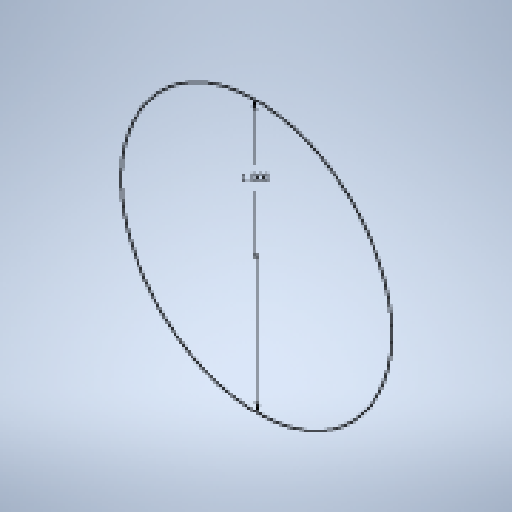
# Autodesk Inventor part: BasePlateMotorMount
Saved by Autodesk Inventor 2023 (Build 270158030, 158C)
## iProperties
Created: 2024-09-27
Part Number: BasePlateMotorMount
Material: Generic
Document SubType Name: Modeling
Designer: lvrectanus0
Density: 1 g/cm^3
Appearance: Default
Author: lvrectanus0
Autodesk Inventor part; units mm, degrees
(part 1 of 2)
ref_plane "YZ Plane" through (0, 0, 0) normal (1, 0, 0) x (0, 1, 0)
ref_plane "XZ Plane" through (0, 0, 0) normal (0, 1, 0) x (-1, 0, 0)
ref_plane "Work Plane1" through (-0.3933, 42.4252, 1.27) normal (0, 0, 1) x (1, 0, 0)
sketch "Sketch2" plane through (-0.3933, 42.4252, 1.27) normal (0, 0, 1) x (1, 0, 0)
  circle A0 centre (0.3933, -42.4252) radius 13.97 projected
  arc A1 (0.495, -45.4235) -> (0.2916, -45.4235) centre (0.3933, -42.4252) ccw projected
  line L0 (0.2916, -45.4235) -> (0.495, -45.4235) projected
  arc A2 (-5.2339, -23.0564) -> (-5.3005, -26.6101) centre (8.4164, -25.0898) ccw projected
  arc A3 (-5.3005, -26.6101) -> (-6.2823, -26.9988) centre (0.3933, -42.4252) ccw projected
  arc A4 (-6.2823, -26.9988) -> (-8.7636, -24.4539) centre (-17.3222, -35.2804) ccw projected
  arc A5 (-8.7636, -24.4539) -> (-9.8739, -25.0643) centre (0.3933, -42.4252) ccw projected
  arc A6 (-9.8739, -25.0643) -> (-9.0547, -28.5229) centre (3.8531, -23.6391) ccw projected
  arc A7 (-9.0547, -28.5229) -> (-9.909, -29.1436) centre (0.3933, -42.4252) ccw projected
  arc A8 (-9.909, -29.1436) -> (-12.9452, -27.2957) centre (-18.5425, -39.9105) ccw projected
  arc A9 (-12.9452, -27.2957) -> (-13.8688, -28.1631) centre (0.3933, -42.4252) ccw projected
  arc A10 (-13.8688, -28.1631) -> (-12.2152, -31.3093) centre (-0.9275, -23.3689) ccw projected
  arc A11 (-12.2152, -31.3093) -> (-12.8883, -32.1229) centre (0.3933, -42.4252) ccw projected
  arc A12 (-12.8883, -32.1229) -> (-16.2887, -31.0882) centre (-18.5729, -44.6986) ccw projected
  arc A13 (-16.2887, -31.0882) -> (-16.9676, -32.158) centre (0.3933, -42.4252) ccw projected
  arc A14 (-16.9676, -32.158) -> (-14.5835, -34.7941) centre (-5.6251, -24.296) ccw projected
  arc A15 (-14.5835, -34.7941) -> (-15.0331, -35.7496) centre (0.3933, -42.4252) ccw projected
  arc A16 (-15.0331, -35.7496) -> (-18.584, -35.593) centre (-17.4117, -49.3439) ccw projected
  arc A17 (-18.584, -35.593) -> (-18.9755, -36.798) centre (0.3933, -42.4252) ccw projected
  arc A18 (-18.9755, -36.798) -> (-16.0107, -38.7585) centre (-9.9445, -26.3623) ccw projected
  arc A19 (-16.0107, -38.7585) -> (-16.2086, -39.7957) centre (0.3933, -42.4252) ccw projected
  arc A20 (-16.2086, -39.7957) -> (-19.6869, -40.5271) centre (-15.1317, -53.5545) ccw projected
  arc A21 (-19.6869, -40.5271) -> (-19.7664, -41.7916) centre (0.3933, -42.4252) ccw projected
  arc A22 (-19.7664, -41.7916) -> (-16.4072, -42.9532) centre (-13.6144, -29.4379) ccw projected
  arc A23 (-16.4072, -42.9532) -> (-16.3409, -44.007) centre (0.3933, -42.4252) ccw projected
  arc A24 (-16.3409, -44.007) -> (-19.5281, -45.5804) centre (-11.8762, -57.0657) ccw projected
  arc A25 (-19.5281, -45.5804) -> (-19.2906, -46.8251) centre (0.3933, -42.4252) ccw projected
  arc A26 (-19.2906, -46.8251) -> (-15.7481, -47.1147) centre (-16.4042, -33.3295) ccw projected
  arc A27 (-15.7481, -47.1147) -> (-15.4218, -48.119) centre (0.3933, -42.4252) ccw projected
  arc A28 (-15.4218, -48.119) -> (-18.1175, -50.4355) centre (-7.8498, -59.6571) ccw projected
  arc A29 (-18.1175, -50.4355) -> (-17.578, -51.582) centre (0.3933, -42.4252) ccw projected
  arc A30 (-17.578, -51.582) -> (-14.0748, -50.9816) centre (-18.1385, -37.7926) ccw projected
  arc A31 (-14.0748, -50.9816) -> (-13.509, -51.8732) centre (0.3933, -42.4252) ccw projected
  arc A32 (-13.509, -51.8732) -> (-15.5439, -54.7873) centre (-3.3054, -61.1657) ccw projected
  arc A33 (-15.5439, -54.7873) -> (-14.7362, -55.7636) centre (0.3933, -42.4252) ccw projected
  arc A34 (-14.7362, -55.7636) -> (-11.4923, -54.3108) centre (-18.7083, -42.5468) ccw projected
  arc A35 (-11.4923, -54.3108) -> (-10.7226, -55.0337) centre (0.3933, -42.4252) ccw projected
  arc A36 (-10.7226, -55.0337) -> (-11.9689, -58.3624) centre (1.4713, -61.4968) ccw projected
  arc A37 (-11.9689, -58.3624) -> (-10.9438, -59.1071) centre (0.3933, -42.4252) ccw projected
  arc A38 (-10.9438, -59.1071) -> (-8.1631, -56.8933) centre (-18.078, -47.2933) ccw projected
  arc A39 (-8.1631, -56.8933) -> (-7.2378, -57.402) centre (0.3933, -42.4252) ccw projected
  arc A40 (-7.2378, -57.402) -> (-7.6171, -60.936) centre (6.1804, -60.6295) ccw projected
  arc A41 (-7.6171, -60.936) -> (-6.439, -61.4025) centre (0.3933, -42.4252) ccw projected
  arc A42 (-6.439, -61.4025) -> (-4.2962, -58.5666) centre (-16.287, -51.734) ccw projected
  arc A43 (-4.2962, -58.5666) -> (-3.2734, -58.8292) centre (0.3933, -42.4252) ccw projected
  arc A44 (-3.2734, -58.8292) -> (-2.7619, -62.3466) centre (10.5258, -58.6184) ccw projected
  arc A45 (-2.7619, -62.3466) -> (-1.5049, -62.5054) centre (0.3933, -42.4252) ccw projected
  arc A46 (-1.5049, -62.5054) -> (-0.1347, -59.2257) centre (-13.448, -55.5898) ccw projected
  arc A47 (-0.1347, -59.2257) -> (0.9213, -59.2257) centre (0.3933, -42.4252) ccw projected
  arc A48 (0.9213, -59.2257) -> (2.2914, -62.5054) centre (14.2345, -55.5898) ccw projected
  arc A49 (2.2914, -62.5054) -> (3.5485, -62.3466) centre (0.3933, -42.4252) ccw projected
  arc A50 (3.5485, -62.3466) -> (4.06, -58.8292) centre (-9.7392, -58.6184) ccw projected
  arc A51 (4.06, -58.8292) -> (5.0828, -58.5666) centre (0.3933, -42.4252) ccw projected
  arc A52 (5.0828, -58.5666) -> (7.2255, -61.4025) centre (17.0736, -51.734) ccw projected
  arc A53 (7.2255, -61.4025) -> (8.4036, -60.936) centre (0.3933, -42.4252) ccw projected
  arc A54 (8.4036, -60.936) -> (8.0243, -57.402) centre (-5.3938, -60.6295) ccw projected
  arc A55 (8.0243, -57.402) -> (8.9497, -56.8933) centre (0.3933, -42.4252) ccw projected
  arc A56 (8.9497, -56.8933) -> (11.7303, -59.1071) centre (18.8646, -47.2933) ccw projected
  arc A57 (11.7303, -59.1071) -> (12.7554, -58.3624) centre (0.3933, -42.4252) ccw projected
  arc A58 (12.7554, -58.3624) -> (11.5092, -55.0337) centre (-0.6848, -61.4968) ccw projected
  arc A59 (11.5092, -55.0337) -> (12.2789, -54.3108) centre (0.3933, -42.4252) ccw projected
  arc A60 (12.2789, -54.3108) -> (15.5228, -55.7636) centre (19.4949, -42.5468) ccw projected
  arc A61 (15.5228, -55.7636) -> (16.3305, -54.7873) centre (0.3933, -42.4252) ccw projected
  arc A62 (16.3305, -54.7873) -> (14.2955, -51.8732) centre (4.092, -61.1657) ccw projected
  arc A63 (14.2955, -51.8732) -> (14.8613, -50.9816) centre (0.3933, -42.4252) ccw projected
  arc A64 (14.8613, -50.9816) -> (18.3646, -51.582) centre (18.925, -37.7926) ccw projected
  arc A65 (18.3646, -51.582) -> (18.9041, -50.4355) centre (0.3933, -42.4252) ccw projected
  arc A66 (18.9041, -50.4355) -> (16.2084, -48.119) centre (8.6364, -59.6571) ccw projected
  arc A67 (16.2084, -48.119) -> (16.5347, -47.1147) centre (0.3933, -42.4252) ccw projected
  arc A68 (16.5347, -47.1147) -> (20.0772, -46.8251) centre (17.1907, -33.3295) ccw projected
  arc A69 (20.0772, -46.8251) -> (20.3146, -45.5804) centre (0.3933, -42.4252) ccw projected
  arc A70 (20.3146, -45.5804) -> (17.1275, -44.007) centre (12.6628, -57.0657) ccw projected
  arc A71 (17.1275, -44.007) -> (17.1938, -42.9532) centre (0.3933, -42.4252) ccw projected
  arc A72 (17.1938, -42.9532) -> (20.553, -41.7916) centre (14.401, -29.4379) ccw projected
  arc A73 (20.553, -41.7916) -> (20.4735, -40.5271) centre (0.3933, -42.4252) ccw projected
  arc A74 (20.4735, -40.5271) -> (16.9952, -39.7957) centre (15.9183, -53.5545) ccw projected
  arc A75 (16.9952, -39.7957) -> (16.7973, -38.7585) centre (0.3933, -42.4252) ccw projected
  arc A76 (16.7973, -38.7585) -> (19.7621, -36.798) centre (10.7311, -26.3623) ccw projected
  arc A77 (19.7621, -36.798) -> (19.3706, -35.593) centre (0.3933, -42.4252) ccw projected
  arc A78 (19.3706, -35.593) -> (15.8197, -35.7496) centre (18.1983, -49.3439) ccw projected
  arc A79 (15.8197, -35.7496) -> (15.3701, -34.7941) centre (0.3933, -42.4252) ccw projected
  arc A80 (15.3701, -34.7941) -> (17.7542, -32.158) centre (6.4116, -24.296) ccw projected
  arc A81 (17.7542, -32.158) -> (17.0752, -31.0882) centre (0.3933, -42.4252) ccw projected
  arc A82 (17.0752, -31.0882) -> (13.6749, -32.1229) centre (19.3595, -44.6986) ccw projected
  arc A83 (13.6749, -32.1229) -> (13.0018, -31.3093) centre (0.3933, -42.4252) ccw projected
  arc A84 (13.0018, -31.3093) -> (14.6554, -28.1631) centre (1.714, -23.3689) ccw projected
  arc A85 (14.6554, -28.1631) -> (13.7317, -27.2957) centre (0.3933, -42.4252) ccw projected
  arc A86 (13.7317, -27.2957) -> (10.6955, -29.1436) centre (19.329, -39.9105) ccw projected
  arc A87 (10.6955, -29.1436) -> (9.8412, -28.5229) centre (0.3933, -42.4252) ccw projected
  arc A88 (9.8412, -28.5229) -> (10.6605, -25.0643) centre (-3.0666, -23.6391) ccw projected
  arc A89 (10.6605, -25.0643) -> (9.5501, -24.4539) centre (0.3933, -42.4252) ccw projected
  arc A90 (9.5501, -24.4539) -> (7.0689, -26.9988) centre (18.1088, -35.2804) ccw projected
  arc A91 (7.0689, -26.9988) -> (6.0871, -26.6101) centre (0.3933, -42.4252) ccw projected
  arc A92 (6.0871, -26.6101) -> (6.0204, -23.0564) centre (-7.6298, -25.0898) ccw projected
  arc A93 (6.0204, -23.0564) -> (4.7932, -22.7413) centre (0.3933, -42.4252) ccw projected
  arc A94 (4.7932, -22.7413) -> (3.0228, -25.8233) centre (15.7754, -31.0992) ccw projected
  arc A95 (3.0228, -25.8233) -> (1.9751, -25.691) centre (0.3933, -42.4252) ccw projected
  arc A96 (1.9751, -25.691) -> (1.0268, -22.2655) centre (-11.6889, -27.6297) ccw projected
  arc A97 (1.0268, -22.2655) -> (-0.2403, -22.2655) centre (0.3933, -42.4252) ccw projected
  arc A98 (-0.2403, -22.2655) -> (-1.1886, -25.691) centre (12.4754, -27.6297) ccw projected
  arc A99 (-1.1886, -25.691) -> (-2.2362, -25.8233) centre (0.3933, -42.4252) ccw projected
  arc A100 (-2.2362, -25.8233) -> (-4.0066, -22.7413) centre (-14.9888, -31.0992) ccw projected
  arc A101 (-4.0066, -22.7413) -> (-5.2339, -23.0564) centre (0.3933, -42.4252) ccw projected
  arc A102 (3.4869, -25.0828) -> (4.2324, -21.6038) centre (-12.0318, -19.9381) ccw projected
  arc A103 (4.2324, -21.6038) -> (5.318, -21.4226) centre (0.3933, 4.7462) ccw projected
  arc A104 (5.318, -21.4226) -> (7.1528, -24.4711) centre (20.1601, -14.5662) ccw projected
  arc A105 (7.1528, -24.4711) -> (8.3544, -24.1668) centre (0.3933, 4.7462) ccw projected
  arc A106 (8.3544, -24.1668) -> (8.5171, -20.6125) centre (-7.7994, -21.6465) ccw projected
  arc A107 (8.5171, -20.6125) -> (9.5581, -20.2551) centre (0.3933, 4.7462) ccw projected
  arc A108 (9.5581, -20.2551) -> (11.8696, -22.9601) centre (23.0692, -11.0493) ccw projected
  arc A109 (11.8696, -22.9601) -> (13.0048, -22.4621) centre (0.3933, 4.7462) ccw projected
  arc A110 (13.0048, -22.4621) -> (12.5802, -18.9295) centre (-3.3436, -22.6351) ccw projected
  arc A111 (12.5802, -18.9295) -> (13.5482, -18.4057) centre (0.3933, 4.7462) ccw projected
  arc A112 (13.5482, -18.4057) -> (16.2734, -20.6932) centre (25.3598, -7.1016) ccw projected
  arc A113 (16.2734, -20.6932) -> (17.3111, -20.0153) centre (0.3933, 4.7462) ccw projected
  arc A114 (17.3111, -20.0153) -> (16.3109, -16.6007) centre (1.2142, -22.8767) ccw projected
  arc A115 (16.3109, -16.6007) -> (17.1795, -15.9247) centre (0.3933, 4.7462) ccw projected
  arc A116 (17.1795, -15.9247) -> (20.244, -17.7325) centre (26.9694, -2.8306) ccw projected
  arc A117 (20.244, -17.7325) -> (21.156, -16.893) centre (0.3933, 4.7462) ccw projected
  arc A118 (21.156, -16.893) -> (19.6074, -13.6896) centre (5.7496, -22.3648) ccw projected
  arc A119 (19.6074, -13.6896) -> (20.3528, -12.8798) centre (0.3933, 4.7462) ccw projected
  arc A120 (20.3528, -12.8798) -> (23.6731, -14.1586) centre (27.854, 1.647) ccw projected
  arc A121 (23.6731, -14.1586) -> (24.4345, -13.1804) centre (0.3933, 4.7462) ccw projected
  arc A122 (24.4345, -13.1804) -> (22.3798, -10.2756) centre (10.1389, -21.1134) ccw projected
  arc A123 (22.3798, -10.2756) -> (22.9818, -9.3542) centre (0.3933, 4.7462) ccw projected
  arc A124 (22.9818, -9.3542) -> (26.4673, -10.069) centre (27.9896, 6.2092) ccw projected
  arc A125 (26.4673, -10.069) -> (27.0572, -8.9789) centre (0.3933, 4.7462) ccw projected
  arc A126 (27.0572, -8.9789) -> (24.5524, -6.4519) centre (14.2623, -19.1567) ccw projected
  arc A127 (24.5524, -6.4519) -> (24.9945, -5.4439) centre (0.3933, 4.7462) ccw projected
  arc A128 (24.9945, -5.4439) -> (28.5502, -5.5753) centre (27.3725, 10.7314) ccw projected
  arc A129 (28.5502, -5.5753) -> (28.9527, -4.4029) centre (0.3933, 4.7462) ccw projected
  arc A130 (28.9527, -4.4029) -> (26.0661, -2.3227) centre (18.0075, -16.5479) ccw projected
  arc A131 (26.0661, -2.3227) -> (26.3363, -1.2557) centre (0.3933, 4.7462) ccw projected
  arc A132 (26.3363, -1.2557) -> (29.865, -0.8001) centre (26.0194, 15.0904) ccw projected
  arc A133 (29.865, -0.8001) -> (30.069, 0.4226) centre (0.3933, 4.7462) ccw projected
  arc A134 (30.069, 0.4226) -> (26.8794, 1.9993) centre (21.2721, -13.3583) ccw projected
  arc A135 (26.8794, 1.9993) -> (26.9703, 3.0962) centre (0.3933, 4.7462) ccw projected
  arc A136 (26.9703, 3.0962) -> (30.376, 4.1265) centre (23.9673, 19.1673) ccw projected
  arc A137 (30.376, 4.1265) -> (30.376, 5.366) centre (0.3933, 4.7462) ccw projected
  arc A138 (30.376, 5.366) -> (26.9703, 6.3963) centre (23.9673, -9.6748) ccw projected
  arc A139 (26.9703, 6.3963) -> (26.8794, 7.4931) centre (0.3933, 4.7462) ccw projected
  arc A140 (26.8794, 7.4931) -> (30.069, 9.0699) centre (21.2721, 22.8507) ccw projected
  arc A141 (30.069, 9.0699) -> (29.865, 10.2925) centre (0.3933, 4.7462) ccw projected
  arc A142 (29.865, 10.2925) -> (26.3363, 10.7482) centre (26.0194, -5.598) ccw projected
  arc A143 (26.3363, 10.7482) -> (26.0661, 11.8152) centre (0.3933, 4.7462) ccw projected
  arc A144 (26.0661, 11.8152) -> (28.9527, 13.8954) centre (18.0075, 26.0404) ccw projected
  arc A145 (28.9527, 13.8954) -> (28.5502, 15.0678) centre (0.3933, 4.7462) ccw projected
  arc A146 (28.5502, 15.0678) -> (24.9945, 14.9364) centre (27.3725, -1.239) ccw projected
  arc A147 (24.9945, 14.9364) -> (24.5524, 15.9444) centre (0.3933, 4.7462) ccw projected
  arc A148 (24.5524, 15.9444) -> (27.0572, 18.4713) centre (14.2623, 28.6491) ccw projected
  arc A149 (27.0572, 18.4713) -> (26.4673, 19.5615) centre (0.3933, 4.7462) ccw projected
  arc A150 (26.4673, 19.5615) -> (22.9818, 18.8467) centre (27.9896, 3.2833) ccw projected
  arc A151 (22.9818, 18.8467) -> (22.3798, 19.7681) centre (0.3933, 4.7462) ccw projected
  arc A152 (22.3798, 19.7681) -> (24.4345, 22.6729) centre (10.1389, 30.6059) ccw projected
  arc A153 (24.4345, 22.6729) -> (23.6731, 23.6511) centre (0.3933, 4.7462) ccw projected
  arc A154 (23.6731, 23.6511) -> (20.3528, 22.3723) centre (27.854, 7.8455) ccw projected
  arc A155 (20.3528, 22.3723) -> (19.6074, 23.1821) centre (0.3933, 4.7462) ccw projected
  arc A156 (19.6074, 23.1821) -> (21.156, 26.3854) centre (5.7496, 31.8573) ccw projected
  arc A157 (21.156, 26.3854) -> (20.244, 27.225) centre (0.3933, 4.7462) ccw projected
  arc A158 (20.244, 27.225) -> (17.1795, 25.4171) centre (26.9694, 12.3231) ccw projected
  arc A159 (17.1795, 25.4171) -> (16.3109, 26.0932) centre (0.3933, 4.7462) ccw projected
  arc A160 (16.3109, 26.0932) -> (17.3111, 29.5077) centre (1.2142, 32.3691) ccw projected
  arc A161 (17.3111, 29.5077) -> (16.2734, 30.1857) centre (0.3933, 4.7462) ccw projected
  arc A162 (16.2734, 30.1857) -> (13.5482, 27.8981) centre (25.3598, 16.594) ccw projected
  arc A163 (13.5482, 27.8981) -> (12.5802, 28.422) centre (0.3933, 4.7462) ccw projected
  arc A164 (12.5802, 28.422) -> (13.0048, 31.9546) centre (-3.3436, 32.1275) ccw projected
  arc A165 (13.0048, 31.9546) -> (11.8696, 32.4525) centre (0.3933, 4.7462) ccw projected
  arc A166 (11.8696, 32.4525) -> (9.5581, 29.7476) centre (23.0692, 20.5418) ccw projected
  arc A167 (9.5581, 29.7476) -> (8.5171, 30.105) centre (0.3933, 4.7462) ccw projected
  arc A168 (8.5171, 30.105) -> (8.3544, 33.6593) centre (-7.7994, 31.139) ccw projected
  arc A169 (8.3544, 33.6593) -> (7.1528, 33.9636) centre (0.3933, 4.7462) ccw projected
  arc A170 (7.1528, 33.9636) -> (5.318, 30.9151) centre (20.1601, 24.0587) ccw projected
  arc A171 (5.318, 30.9151) -> (4.2324, 31.0962) centre (0.3933, 4.7462) ccw projected
  arc A172 (4.2324, 31.0962) -> (3.4869, 34.5753) centre (-12.0318, 29.4306) ccw projected
  arc A173 (3.4869, 34.5753) -> (2.2516, 34.6777) centre (0.3933, 4.7462) ccw projected
  arc A174 (2.2516, 34.6777) -> (0.9436, 31.3688) centre (16.7118, 27.0488) ccw projected
  arc A175 (0.9436, 31.3688) -> (-0.157, 31.3688) centre (0.3933, 4.7462) ccw projected
  arc A176 (-0.157, 31.3688) -> (-1.465, 34.6777) centre (-15.9252, 27.0488) ccw projected
  arc A177 (-1.465, 34.6777) -> (-2.7003, 34.5753) centre (0.3933, 4.7462) ccw projected
  arc A178 (-2.7003, 34.5753) -> (-3.4458, 31.0962) centre (12.8183, 29.4306) ccw projected
  arc A179 (-3.4458, 31.0962) -> (-4.5315, 30.9151) centre (0.3933, 4.7462) ccw projected
  arc A180 (-4.5315, 30.9151) -> (-6.3662, 33.9636) centre (-19.3735, 24.0587) ccw projected
  arc A181 (-6.3662, 33.9636) -> (-7.5678, 33.6593) centre (0.3933, 4.7462) ccw projected
  arc A182 (-7.5678, 33.6593) -> (-7.7305, 30.105) centre (8.586, 31.139) ccw projected
  arc A183 (-7.7305, 30.105) -> (-8.7715, 29.7476) centre (0.3933, 4.7462) ccw projected
  arc A184 (-8.7715, 29.7476) -> (-11.083, 32.4525) centre (-22.2827, 20.5418) ccw projected
  arc A185 (-11.083, 32.4525) -> (-12.2182, 31.9546) centre (0.3933, 4.7462) ccw projected
  arc A186 (-12.2182, 31.9546) -> (-11.7936, 28.422) centre (4.1301, 32.1275) ccw projected
  arc A187 (-11.7936, 28.422) -> (-12.7616, 27.8981) centre (0.3933, 4.7462) ccw projected
  arc A188 (-12.7616, 27.8981) -> (-15.4868, 30.1857) centre (-24.5733, 16.594) ccw projected
  arc A189 (-15.4868, 30.1857) -> (-16.5245, 29.5077) centre (0.3933, 4.7462) ccw projected
  arc A190 (-16.5245, 29.5077) -> (-15.5243, 26.0932) centre (-0.4277, 32.3691) ccw projected
  arc A191 (-15.5243, 26.0932) -> (-16.3929, 25.4171) centre (0.3933, 4.7462) ccw projected
  arc A192 (-16.3929, 25.4171) -> (-19.4574, 27.225) centre (-26.1828, 12.3231) ccw projected
  arc A193 (-19.4574, 27.225) -> (-20.3694, 26.3854) centre (0.3933, 4.7462) ccw projected
  arc A194 (-20.3694, 26.3854) -> (-18.8208, 23.1821) centre (-4.963, 31.8573) ccw projected
  arc A195 (-18.8208, 23.1821) -> (-19.5663, 22.3723) centre (0.3933, 4.7462) ccw projected
  arc A196 (-19.5663, 22.3723) -> (-22.8866, 23.6511) centre (-27.0675, 7.8455) ccw projected
  arc A197 (-22.8866, 23.6511) -> (-23.6479, 22.6729) centre (0.3933, 4.7462) ccw projected
  arc A198 (-23.6479, 22.6729) -> (-21.5932, 19.7681) centre (-9.3523, 30.6059) ccw projected
  arc A199 (-21.5932, 19.7681) -> (-22.1952, 18.8467) centre (0.3933, 4.7462) ccw projected
  arc A200 (-22.1952, 18.8467) -> (-25.6807, 19.5615) centre (-27.2031, 3.2833) ccw projected
  arc A201 (-25.6807, 19.5615) -> (-26.2707, 18.4713) centre (0.3933, 4.7462) ccw projected
  arc A202 (-26.2707, 18.4713) -> (-23.7659, 15.9444) centre (-13.4758, 28.6491) ccw projected
  arc A203 (-23.7659, 15.9444) -> (-24.208, 14.9364) centre (0.3933, 4.7462) ccw projected
  arc A204 (-24.208, 14.9364) -> (-27.7636, 15.0678) centre (-26.5859, -1.239) ccw projected
  arc A205 (-27.7636, 15.0678) -> (-28.1661, 13.8954) centre (0.3933, 4.7462) ccw projected
  arc A206 (-28.1661, 13.8954) -> (-25.2795, 11.8152) centre (-17.2209, 26.0404) ccw projected
  arc A207 (-25.2795, 11.8152) -> (-25.5497, 10.7482) centre (0.3933, 4.7462) ccw projected
  arc A208 (-25.5497, 10.7482) -> (-29.0784, 10.2925) centre (-25.2328, -5.598) ccw projected
  arc A209 (-29.0784, 10.2925) -> (-29.2825, 9.0699) centre (0.3933, 4.7462) ccw projected
  arc A210 (-29.2825, 9.0699) -> (-26.0929, 7.4931) centre (-20.4856, 22.8507) ccw projected
  arc A211 (-26.0929, 7.4931) -> (-26.1838, 6.3963) centre (0.3933, 4.7462) ccw projected
  arc A212 (-26.1838, 6.3963) -> (-29.5894, 5.366) centre (-23.1807, -9.6748) ccw projected
  arc A213 (-29.5894, 5.366) -> (-29.5894, 4.1265) centre (0.3933, 4.7462) ccw projected
  arc A214 (-29.5894, 4.1265) -> (-26.1838, 3.0962) centre (-23.1807, 19.1673) ccw projected
  arc A215 (-26.1838, 3.0962) -> (-26.0929, 1.9993) centre (0.3933, 4.7462) ccw projected
  arc A216 (-26.0929, 1.9993) -> (-29.2825, 0.4226) centre (-20.4856, -13.3583) ccw projected
  arc A217 (-29.2825, 0.4226) -> (-29.0784, -0.8001) centre (0.3933, 4.7462) ccw projected
  arc A218 (-29.0784, -0.8001) -> (-25.5497, -1.2557) centre (-25.2328, 15.0904) ccw projected
  arc A219 (-25.5497, -1.2557) -> (-25.2795, -2.3227) centre (0.3933, 4.7462) ccw projected
  arc A220 (-25.2795, -2.3227) -> (-28.1661, -4.4029) centre (-17.2209, -16.5479) ccw projected
  arc A221 (-28.1661, -4.4029) -> (-27.7636, -5.5753) centre (0.3933, 4.7462) ccw projected
  arc A222 (-27.7636, -5.5753) -> (-24.208, -5.4439) centre (-26.5859, 10.7314) ccw projected
  arc A223 (-24.208, -5.4439) -> (-23.7659, -6.4519) centre (0.3933, 4.7462) ccw projected
  arc A224 (-23.7659, -6.4519) -> (-26.2707, -8.9789) centre (-13.4758, -19.1567) ccw projected
  arc A225 (-26.2707, -8.9789) -> (-25.6807, -10.069) centre (0.3933, 4.7462) ccw projected
  arc A226 (-25.6807, -10.069) -> (-22.1952, -9.3542) centre (-27.2031, 6.2092) ccw projected
  arc A227 (-22.1952, -9.3542) -> (-21.5932, -10.2756) centre (0.3933, 4.7462) ccw projected
  arc A228 (-21.5932, -10.2756) -> (-23.6479, -13.1804) centre (-9.3523, -21.1134) ccw projected
  arc A229 (-23.6479, -13.1804) -> (-22.8866, -14.1586) centre (0.3933, 4.7462) ccw projected
  arc A230 (-22.8866, -14.1586) -> (-19.5663, -12.8798) centre (-27.0675, 1.647) ccw projected
  arc A231 (-19.5663, -12.8798) -> (-18.8208, -13.6896) centre (0.3933, 4.7462) ccw projected
  arc A232 (-18.8208, -13.6896) -> (-20.3694, -16.893) centre (-4.963, -22.3648) ccw projected
  arc A233 (-20.3694, -16.893) -> (-19.4574, -17.7325) centre (0.3933, 4.7462) ccw projected
  arc A234 (-19.4574, -17.7325) -> (-16.3929, -15.9247) centre (-26.1828, -2.8306) ccw projected
  arc A235 (-16.3929, -15.9247) -> (-15.5243, -16.6007) centre (0.3933, 4.7462) ccw projected
  arc A236 (-15.5243, -16.6007) -> (-16.5245, -20.0153) centre (-0.4277, -22.8767) ccw projected
  arc A237 (-16.5245, -20.0153) -> (-15.4868, -20.6932) centre (0.3933, 4.7462) ccw projected
  arc A238 (-15.4868, -20.6932) -> (-12.7616, -18.4057) centre (-24.5733, -7.1016) ccw projected
  arc A239 (-12.7616, -18.4057) -> (-11.7936, -18.9295) centre (0.3933, 4.7462) ccw projected
  arc A240 (-11.7936, -18.9295) -> (-12.2182, -22.4621) centre (4.1301, -22.6351) ccw projected
  arc A241 (-12.2182, -22.4621) -> (-11.083, -22.9601) centre (0.3933, 4.7462) ccw projected
  arc A242 (-11.083, -22.9601) -> (-8.7715, -20.2551) centre (-22.2827, -11.0493) ccw projected
  arc A243 (-8.7715, -20.2551) -> (-7.7305, -20.6125) centre (0.3933, 4.7462) ccw projected
  arc A244 (-7.7305, -20.6125) -> (-7.5678, -24.1668) centre (8.586, -21.6465) ccw projected
  arc A245 (-7.5678, -24.1668) -> (-6.3662, -24.4711) centre (0.3933, 4.7462) ccw projected
  arc A246 (-6.3662, -24.4711) -> (-4.5315, -21.4226) centre (-19.3735, -14.5662) ccw projected
  arc A247 (-4.5315, -21.4226) -> (-3.4458, -21.6038) centre (0.3933, 4.7462) ccw projected
  arc A248 (-3.4458, -21.6038) -> (-2.7003, -25.0828) centre (12.8183, -19.9381) ccw projected
  arc A249 (-2.7003, -25.0828) -> (-1.465, -25.1852) centre (0.3933, 4.7462) ccw projected
  arc A250 (-1.465, -25.1852) -> (-0.157, -21.8763) centre (-15.9252, -17.5564) ccw projected
  arc A251 (-0.157, -21.8763) -> (0.9436, -21.8763) centre (0.3933, 4.7462) ccw projected
  arc A252 (0.9436, -21.8763) -> (2.2516, -25.1852) centre (16.7118, -17.5564) ccw projected
  arc A253 (2.2516, -25.1852) -> (3.4869, -25.0828) centre (0.3933, 4.7462) ccw projected
  line L1 (3.3661, -1.5533) -> (7.3352, 4.171) projected
  line L2 (-3.5758, -0.978) -> (3.3661, -1.5533) projected
  line L3 (-6.5487, 5.3215) -> (-3.5758, -0.978) projected
  line L4 (-2.5795, 11.0457) -> (-6.5487, 5.3215) projected
  line L5 (4.3624, 10.4705) -> (-2.5795, 11.0457) projected
  line L6 (7.3352, 4.171) -> (4.3624, 10.4705) projected
  arc A254 (5.8315, -120.0023) -> (6.7501, -116.5589) centre (-13.9026, -112.8937) ccw projected
  arc A255 (4.6244, -120.0775) -> (5.8315, -120.0023) centre (0.3933, -42.4252) ccw projected
  arc A256 (3.2855, -116.7747) -> (4.6244, -120.0775) centre (23.3237, -110.5748) ccw projected
  arc A257 (2.1289, -116.8107) -> (3.2855, -116.7747) centre (0.3933, -42.4252) ccw projected
  arc A258 (0.998, -120.1904) -> (2.1289, -116.8107) centre (-18.256, -111.8686) ccw projected
  arc A259 (-0.2114, -120.1904) -> (0.998, -120.1904) centre (0.3933, -42.4252) ccw projected
  arc A260 (-1.3423, -116.8107) -> (-0.2114, -120.1904) centre (19.0425, -111.8686) ccw projected
  arc A261 (-2.499, -116.7747) -> (-1.3423, -116.8107) centre (0.3933, -42.4252) ccw projected
  arc A262 (-3.8378, -120.0775) -> (-2.499, -116.7747) centre (-22.5371, -110.5748) ccw projected
  arc A263 (-5.0449, -120.0023) -> (-3.8378, -120.0775) centre (0.3933, -42.4252) ccw projected
  arc A264 (-5.9635, -116.5589) -> (-5.0449, -120.0023) centre (14.6892, -112.8937) ccw projected
  arc A265 (-7.1157, -116.4511) -> (-5.9635, -116.5589) centre (0.3933, -42.4252) ccw projected
  arc A266 (-8.6572, -119.6643) -> (-7.1157, -116.4511) centre (-26.7296, -109.0174) ccw projected
  arc A267 (-9.8573, -119.5142) -> (-8.6572, -119.6643) centre (0.3933, -42.4252) ccw projected
  arc A268 (-10.5601, -116.0203) -> (-9.8573, -119.5142) centre (10.2805, -113.6461) ccw projected
  arc A269 (-11.7033, -115.8411) -> (-10.5601, -116.0203) centre (0.3933, -42.4252) ccw projected
  arc A270 (-13.4416, -118.9522) -> (-11.7033, -115.8411) centre (-30.8172, -107.2024) ccw projected
  arc A271 (-14.6301, -118.7278) -> (-13.4416, -118.9522) centre (0.3933, -42.4252) ccw projected
  arc A272 (-15.1143, -115.197) -> (-14.6301, -118.7278) centre (5.8336, -114.123) ccw projected
  arc A273 (-16.2441, -114.947) -> (-15.1143, -115.197) centre (0.3933, -42.4252) ccw projected
  arc A274 (-18.1725, -117.944) -> (-16.2441, -114.947) centre (-34.784, -105.1367) ccw projected
  arc A275 (-19.3447, -117.6462) -> (-18.1725, -117.944) centre (0.3933, -42.4252) ccw projected
  arc A276 (-19.6085, -114.0921) -> (-19.3447, -117.6462) centre (1.3657, -114.3226) ccw projected
  arc A277 (-20.7206, -113.7724) -> (-19.6085, -114.0921) centre (0.3933, -42.4252) ccw projected
  arc A278 (-22.8316, -116.6437) -> (-20.7206, -113.7724) centre (-38.6147, -102.8285) ccw projected
  arc A279 (-23.983, -116.2736) -> (-22.8316, -116.6437) centre (0.3933, -42.4252) ccw projected
  arc A280 (-24.0253, -112.71) -> (-23.983, -116.2736) centre (-3.106, -114.2439) ccw projected
  arc A281 (-25.1154, -112.3217) -> (-24.0253, -112.71) centre (0.3933, -42.4252) ccw projected
  arc A282 (-27.4008, -115.0563) -> (-25.1154, -112.3217) centre (-42.2945, -100.2865) ccw projected
  arc A283 (-28.527, -114.6152) -> (-27.4008, -115.0563) centre (0.3933, -42.4252) ccw projected
  arc A284 (-28.3476, -111.0559) -> (-28.527, -114.6152) centre (-7.5642, -113.8875) ccw projected
  arc A285 (-29.4115, -110.6006) -> (-28.3476, -111.0559) centre (0.3933, -42.4252) ccw projected
  arc A286 (-31.8625, -113.1878) -> (-29.4115, -110.6006) centre (-45.8091, -97.5207) ccw projected
  arc A287 (-32.9591, -112.6776) -> (-31.8625, -113.1878) centre (0.3933, -42.4252) ccw projected
  arc A288 (-32.5588, -109.1363) -> (-32.9591, -112.6776) centre (-11.9916, -113.2545) ccw projected
  arc A289 (-33.5923, -108.6158) -> (-32.5588, -109.1363) centre (0.3933, -42.4252) ccw projected
  arc A290 (-36.1994, -111.0456) -> (-33.5923, -108.6158) centre (-49.145, -94.5417) ccw projected
  arc A291 (-37.2621, -110.4682) -> (-36.1994, -111.0456) centre (0.3933, -42.4252) ccw projected
  arc A292 (-36.6424, -106.9587) -> (-37.2621, -110.4682) centre (-16.3711, -112.3475) ccw projected
  arc A293 (-37.6416, -106.3749) -> (-36.6424, -106.9587) centre (0.3933, -42.4252) ccw projected
  arc A294 (-40.3947, -108.6379) -> (-37.6416, -106.3749) centre (-52.2893, -91.3612) ccw projected
  arc A295 (-41.4195, -107.9956) -> (-40.3947, -108.6379) centre (0.3933, -42.4252) ccw projected
  arc A296 (-40.5828, -104.5313) -> (-41.4195, -107.9956) centre (-20.6857, -111.17) ccw projected
  arc A297 (-41.5437, -103.8866) -> (-40.5828, -104.5313) centre (0.3933, -42.4252) ccw projected
  arc A298 (-44.4322, -105.9741) -> (-41.5437, -103.8866) centre (-55.2297, -87.9912) ccw projected
  arc A299 (-45.4151, -105.2693) -> (-44.4322, -105.9741) centre (0.3933, -42.4252) ccw projected
  arc A300 (-44.3647, -101.8637) -> (-45.4151, -105.2693) centre (-24.9188, -109.7266) ccw projected
  arc A301 (-45.2836, -101.1605) -> (-44.3647, -101.8637) centre (0.3933, -42.4252) ccw projected
  arc A302 (-48.2963, -103.0644) -> (-45.2836, -101.1605) centre (-57.9549, -84.445) ccw projected
  arc A303 (-49.2335, -102.2998) -> (-48.2963, -103.0644) centre (0.3933, -42.4252) ccw projected
  arc A304 (-47.9734, -98.9662) -> (-49.2335, -102.2998) centre (-29.0539, -108.0228) ccw projected
  arc A305 (-48.8468, -98.2072) -> (-47.9734, -98.9662) centre (0.3933, -42.4252) ccw projected
  arc A306 (-51.9721, -99.92) -> (-48.8468, -98.2072) centre (-60.4544, -80.7363) ccw projected
  arc A307 (-52.8599, -99.0987) -> (-51.9721, -99.92) centre (0.3933, -42.4252) ccw projected
  arc A308 (-51.3949, -95.8499) -> (-52.8599, -99.0987) centre (-33.0751, -106.0651) ccw projected
  arc A309 (-52.2195, -95.038) -> (-51.3949, -95.8499) centre (0.3933, -42.4252) ccw projected
  arc A310 (-55.4452, -96.5533) -> (-52.2195, -95.038) centre (-62.7185, -76.8793) ccw projected
  arc A311 (-56.2802, -95.6784) -> (-55.4452, -96.5533) centre (0.3933, -42.4252) ccw projected
  arc A312 (-54.6162, -92.5269) -> (-56.2802, -95.6784) centre (-36.9669, -103.8613) ccw projected
  arc A313 (-55.3887, -91.6653) -> (-54.6162, -92.5269) centre (0.3933, -42.4252) ccw projected
  arc A314 (-58.7023, -92.9771) -> (-55.3887, -91.6653) centre (-64.7384, -72.889) ccw projected
  arc A315 (-59.4813, -92.052) -> (-58.7023, -92.9771) centre (0.3933, -42.4252) ccw projected
  arc A316 (-57.6245, -89.01) -> (-59.4813, -92.052) centre (-40.7141, -101.4198) ccw projected
  arc A317 (-58.342, -88.1021) -> (-57.6245, -89.01) centre (0.3933, -42.4252) ccw projected
  arc A318 (-61.7308, -89.2054) -> (-58.342, -88.1021) centre (-66.5063, -68.7809) ccw projected
  arc A319 (-62.4508, -88.2336) -> (-61.7308, -89.2054) centre (0.3933, -42.4252) ccw projected
  arc A320 (-60.4085, -85.313) -> (-62.4508, -88.2336) centre (-44.3022, -98.7501) ccw projected
  arc A321 (-61.0681, -84.3622) -> (-60.4085, -85.313) centre (0.3933, -42.4252) ccw projected
  arc A322 (-64.5189, -85.2527) -> (-61.0681, -84.3622) centre (-68.0154, -64.5707) ccw projected
  arc A323 (-65.1771, -84.238) -> (-64.5189, -85.2527) centre (0.3933, -42.4252) ccw projected
  arc A324 (-62.9572, -81.45) -> (-65.1771, -84.238) centre (-47.7174, -95.8624) ccw projected
  arc A325 (-63.5564, -80.4601) -> (-62.9572, -81.45) centre (0.3933, -42.4252) ccw projected
  arc A326 (-67.0559, -81.1342) -> (-63.5564, -80.4601) centre (-69.2599, -60.275) ccw projected
  arc A327 (-67.6498, -80.0806) -> (-67.0559, -81.1342) centre (0.3933, -42.4252) ccw projected
  arc A328 (-65.2608, -77.436) -> (-67.6498, -80.0806) centre (-50.9466, -92.768) ccw projected
  arc A329 (-65.7973, -76.4107) -> (-65.2608, -77.436) centre (0.3933, -42.4252) ccw projected
  arc A330 (-69.332, -76.8661) -> (-65.7973, -76.4107) centre (-70.2349, -55.9101) ccw projected
  arc A331 (-69.8592, -75.7776) -> (-69.332, -76.8661) centre (0.3933, -42.4252) ccw projected
  arc A332 (-67.3104, -73.2866) -> (-69.8592, -75.7776) centre (-53.977, -89.4788) ccw projected
  arc A333 (-67.7822, -72.23) -> (-67.3104, -73.2866) centre (0.3933, -42.4252) ccw projected
  arc A334 (-71.3383, -72.4647) -> (-67.7822, -72.23) centre (-70.9366, -51.4931) ccw projected
  arc A335 (-71.7968, -71.3455) -> (-71.3383, -72.4647) centre (0.3933, -42.4252) ccw projected
  arc A336 (-69.0981, -69.0178) -> (-71.7968, -71.3455) centre (-56.7972, -86.0076) ccw projected
  arc A337 (-69.5032, -67.9339) -> (-69.0981, -69.0178) centre (0.3933, -42.4252) ccw projected
  arc A338 (-73.0671, -67.947) -> (-69.5032, -67.9339) centre (-71.3624, -47.041) ccw projected
  arc A339 (-73.4551, -66.8015) -> (-73.0671, -67.947) centre (0.3933, -42.4252) ccw projected
  arc A340 (-70.6169, -64.6461) -> (-73.4551, -66.8015) centre (-59.396, -82.3678) ccw projected
  arc A341 (-70.9539, -63.5391) -> (-70.6169, -64.6461) centre (0.3933, -42.4252) ccw projected
  arc A342 (-74.5116, -63.3307) -> (-70.9539, -63.5391) centre (-71.5105, -42.5711) ccw projected
  arc A343 (-74.8277, -62.1632) -> (-74.5116, -63.3307) centre (0.3933, -42.4252) ccw projected
  arc A344 (-71.861, -60.1884) -> (-74.8277, -62.1632) centre (-61.7636, -78.5735) ccw projected
  arc A345 (-72.1285, -59.0626) -> (-71.861, -60.1884) centre (0.3933, -42.4252) ccw projected
  arc A346 (-75.6664, -58.6334) -> (-72.1285, -59.0626) centre (-71.3805, -38.1006) ccw projected
  arc A347 (-75.9093, -57.4486) -> (-75.6664, -58.6334) centre (0.3933, -42.4252) ccw projected
  arc A348 (-72.8256, -55.6621) -> (-75.9093, -57.4486) centre (-63.8907, -74.6393) ccw projected
  arc A349 (-73.0226, -54.5218) -> (-72.8256, -55.6621) centre (0.3933, -42.4252) ccw projected
  arc A350 (-76.527, -53.8734) -> (-73.0226, -54.5218) centre (-70.9728, -33.6468) ccw projected
  arc A351 (-76.6957, -52.6758) -> (-76.527, -53.8734) centre (0.3933, -42.4252) ccw projected
  arc A352 (-73.5069, -51.0845) -> (-76.6957, -52.6758) centre (-65.7691, -70.5805) ccw projected
  arc A353 (-73.6326, -49.9341) -> (-73.5069, -51.0845) centre (0.3933, -42.4252) ccw projected
  arc A354 (-77.0899, -49.0692) -> (-73.6326, -49.9341) centre (-70.289, -29.2269) ccw projected
  arc A355 (-77.1839, -47.8634) -> (-77.0899, -49.0692) centre (0.3933, -42.4252) ccw projected
  arc A356 (-73.9023, -46.4734) -> (-77.1839, -47.8634) centre (-67.3915, -66.4127) ccw projected
  arc A357 (-73.9562, -45.3174) -> (-73.9023, -46.4734) centre (0.3933, -42.4252) ccw projected
  arc A358 (-77.3531, -44.2392) -> (-73.9562, -45.3174) centre (-69.3317, -24.8582) ccw projected
  arc A359 (-77.3719, -43.0299) -> (-77.3531, -44.2392) centre (0.3933, -42.4252) ccw projected
  arc A360 (-74.0102, -41.8466) -> (-77.3719, -43.0299) centre (-68.7517, -62.1521) ccw projected
  arc A361 (-73.9922, -40.6896) -> (-74.0102, -41.8466) centre (0.3933, -42.4252) ccw projected
  arc A362 (-77.3155, -39.4023) -> (-73.9922, -40.6896) centre (-68.1047, -20.5574) ccw projected
  arc A363 (-77.259, -38.1941) -> (-77.3155, -39.4023) centre (0.3933, -42.4252) ccw projected
  arc A364 (-73.8303, -37.2221) -> (-77.259, -38.1941) centre (-69.8443, -57.8153) ccw projected
  arc A365 (-73.7404, -36.0684) -> (-73.8303, -37.2221) centre (0.3933, -42.4252) ccw projected
  arc A366 (-76.9772, -34.577) -> (-73.7404, -36.0684) centre (-66.6127, -16.3412) ccw projected
  arc A367 (-76.8458, -33.3747) -> (-76.9772, -34.577) centre (0.3933, -42.4252) ccw projected
  arc A368 (-73.3633, -32.6177) -> (-76.8458, -33.3747) centre (-70.6653, -53.4189) ccw projected
  arc A369 (-73.2018, -31.4718) -> (-73.3633, -32.6177) centre (0.3933, -42.4252) ccw projected
  arc A370 (-76.3396, -29.7821) -> (-73.2018, -31.4718) centre (-64.8615, -12.2259) ccw projected
  arc A371 (-76.1337, -28.5903) -> (-76.3396, -29.7821) centre (0.3933, -42.4252) ccw projected
  arc A372 (-72.6109, -28.0512) -> (-76.1337, -28.5903) centre (-71.2113, -48.9799) ccw projected
  arc A373 (-72.3785, -26.9176) -> (-72.6109, -28.0512) centre (0.3933, -42.4252) ccw projected
  arc A374 (-75.4052, -25.0361) -> (-72.3785, -26.9176) centre (-62.8577, -8.2275) ccw projected
  arc A375 (-75.1256, -23.8594) -> (-75.4052, -25.0361) centre (0.3933, -42.4252) ccw projected
  arc A376 (-71.576, -23.5404) -> (-75.1256, -23.8594) centre (-71.4803, -44.5156) ccw projected
  arc A377 (-71.2736, -22.4234) -> (-71.576, -23.5404) centre (0.3933, -42.4252) ccw projected
  arc A378 (-74.1775, -20.3574) -> (-71.2736, -22.4234) centre (-60.6093, -4.3613) ccw projected
  arc A379 (-73.8253, -19.2003) -> (-74.1775, -20.3574) centre (0.3933, -42.4252) ccw projected
  arc A380 (-70.2627, -19.1026) -> (-73.8253, -19.2003) centre (-71.4712, -40.0432) ccw projected
  arc A381 (-69.8915, -18.0066) -> (-70.2627, -19.1026) centre (0.3933, -42.4252) ccw projected
  arc A382 (-72.6613, -15.764) -> (-69.8915, -18.0066) centre (-58.1249, -0.6424) ccw projected
  arc A383 (-72.2378, -14.6311) -> (-72.6613, -15.764) centre (0.3933, -42.4252) ccw projected
  arc A384 (-68.6761, -14.7551) -> (-72.2378, -14.6311) centre (-71.1841, -35.58) ccw projected
  arc A385 (-68.2374, -13.6843) -> (-68.6761, -14.7551) centre (0.3933, -42.4252) ccw projected
  arc A386 (-70.8624, -11.2738) -> (-68.2374, -13.6843) centre (-55.4141, 2.9148) ccw projected
  arc A387 (-70.3694, -10.1694) -> (-70.8624, -11.2738) centre (0.3933, -42.4252) ccw projected
  arc A388 (-66.8223, -10.5146) -> (-70.3694, -10.1694) centre (-70.6201, -31.1433) ccw projected
  arc A389 (-66.3179, -9.4731) -> (-66.8223, -10.5146) centre (0.3933, -42.4252) ccw projected
  arc A390 (-68.7879, -6.9041) -> (-66.3179, -9.4731) centre (-52.4874, 6.2966) ccw projected
  arc A391 (-68.2271, -5.8325) -> (-68.7879, -6.9041) centre (0.3933, -42.4252) ccw projected
  arc A392 (-64.7084, -6.3976) -> (-68.2271, -5.8325) centre (-69.7813, -26.7503) ccw projected
  arc A393 (-64.1402, -5.3895) -> (-64.7084, -6.3976) centre (0.3933, -42.4252) ccw projected
  arc A394 (-66.4458, -2.6719) -> (-64.1402, -5.3895) centre (-49.3561, 9.4899) ccw projected
  arc A395 (-65.8195, -1.6372) -> (-66.4458, -2.6719) centre (0.3933, -42.4252) ccw projected
  arc A396 (-62.3426, -2.4199) -> (-65.8195, -1.6372) centre (-68.6711, -22.4179) ccw projected
  arc A397 (-61.7129, -1.4491) -> (-62.3426, -2.4199) centre (0.3933, -42.4252) ccw projected
  arc A398 (-63.845, 1.4066) -> (-61.7129, -1.4491) centre (-46.0323, 12.4824) ccw projected
  arc A399 (-63.1556, 2.4003) -> (-63.845, 1.4066) centre (0.3933, -42.4252) ccw projected
  arc A400 (-59.7341, 1.403) -> (-63.1556, 2.4003) centre (-67.2936, -18.1629) ccw projected
  arc A401 (-59.0453, 2.3328) -> (-59.7341, 1.403) centre (0.3933, -42.4252) ccw projected
  arc A402 (-60.9958, 5.3155) -> (-59.0453, 2.3328) centre (-42.5289, 15.2625) ccw projected
  arc A403 (-60.2459, 6.2644) -> (-60.9958, 5.3155) centre (0.3933, -42.4252) ccw projected
  arc A404 (-56.893, 5.0563) -> (-60.2459, 6.2644) centre (-65.6543, -14.0017) ccw projected
  arc A405 (-56.1477, 5.9415) -> (-56.893, 5.0563) centre (0.3933, -42.4252) ccw projected
  arc A406 (-57.909, 9.0397) -> (-56.1477, 5.9415) centre (-38.8594, 17.8193) ccw projected
  arc A407 (-57.1016, 9.9401) -> (-57.909, 9.0397) centre (0.3933, -42.4252) ccw projected
  arc A408 (-53.8303, 8.5259) -> (-57.1016, 9.9401) centre (-63.7595, -9.9505) ccw projected
  arc A409 (-53.0314, 9.363) -> (-53.8303, 8.5259) centre (0.3933, -42.4252) ccw projected
  arc A410 (-54.5967, 12.5647) -> (-53.0314, 9.363) centre (-35.0381, 20.1431) ccw projected
  arc A411 (-53.7348, 13.4133) -> (-54.5967, 12.5647) centre (0.3933, -42.4252) ccw projected
  arc A412 (-50.5578, 11.7984) -> (-53.7348, 13.4133) centre (-61.6164, -6.025) ccw projected
  arc A413 (-49.7084, 12.5842) -> (-50.5578, 11.7984) centre (0.3933, -42.4252) ccw projected
  arc A414 (-51.0716, 15.8771) -> (-49.7084, 12.5842) centre (-31.0797, 22.2248) ccw projected
  arc A415 (-50.1586, 16.6704) -> (-51.0716, 15.8771) centre (0.3933, -42.4252) ccw projected
  arc A416 (-47.0882, 14.8611) -> (-50.1586, 16.6704) centre (-59.2335, -2.2403) ccw projected
  arc A417 (-46.1916, 15.5926) -> (-47.0882, 14.8611) centre (0.3933, -42.4252) ccw projected
  arc A418 (-47.3474, 18.9638) -> (-46.1916, 15.5926) centre (-26.9996, 24.0564) ccw projected
  arc A419 (-46.3869, 19.6989) -> (-47.3474, 18.9638) centre (0.3933, -42.4252) ccw projected
  arc A420 (-43.4349, 17.7022) -> (-46.3869, 19.6989) centre (-56.6199, 1.3889) ccw projected
  arc A421 (-42.4945, 18.3766) -> (-43.4349, 17.7022) centre (0.3933, -42.4252) ccw projected
  arc A422 (-43.4385, 21.8131) -> (-42.4945, 18.3766) centre (-22.8135, 25.6308) ccw projected
  arc A423 (-42.4342, 22.487) -> (-43.4385, 21.8131) centre (0.3933, -42.4252) ccw projected
  arc A424 (-39.612, 20.3107) -> (-42.4342, 22.487) centre (-53.7857, 4.8487) ccw projected
  arc A425 (-38.6315, 20.9253) -> (-39.612, 20.3107) centre (0.3933, -42.4252) ccw projected
  arc A426 (-39.36, 24.4139) -> (-38.6315, 20.9253) centre (-18.5376, 26.942) ccw projected
  arc A427 (-38.3158, 25.024) -> (-39.36, 24.4139) centre (0.3933, -42.4252) ccw projected
  arc A428 (-35.6343, 22.6765) -> (-38.3158, 25.024) centre (-50.7419, 8.1255) ccw projected
  arc A429 (-34.6175, 23.2289) -> (-35.6343, 22.6765) centre (0.3933, -42.4252) ccw projected
  arc A430 (-35.1278, 26.756) -> (-34.6175, 23.2289) centre (-14.1884, 27.9847) ccw projected
  arc A431 (-34.0476, 27.3001) -> (-35.1278, 26.756) centre (0.3933, -42.4252) ccw projected
  arc A432 (-31.5173, 24.7904) -> (-34.0476, 27.3001) centre (-47.5002, 11.2068) ccw projected
  arc A433 (-30.4681, 25.2785) -> (-31.5173, 24.7904) centre (0.3933, -42.4252) ccw projected
  arc A434 (-30.7581, 28.8305) -> (-30.4681, 25.2785) centre (-9.7828, 28.755) ccw projected
  arc A435 (-29.6462, 29.3064) -> (-30.7581, 28.8305) centre (0.3933, -42.4252) ccw projected
  arc A436 (-27.2768, 26.6442) -> (-29.6462, 29.3064) centre (-44.0733, 14.0806) ccw projected
  arc A437 (-26.1993, 27.0662) -> (-27.2768, 26.6442) centre (0.3933, -42.4252) ccw projected
  arc A438 (-26.2679, 30.6294) -> (-26.1993, 27.0662) centre (-5.3379, 29.25) ccw projected
  arc A439 (-25.1285, 31.0352) -> (-26.2679, 30.6294) centre (0.3933, -42.4252) ccw projected
  arc A440 (-22.9293, 28.2308) -> (-25.1285, 31.0352) centre (-40.4743, 16.7357) ccw projected
  arc A441 (-21.8276, 28.585) -> (-22.9293, 28.2308) centre (0.3933, -42.4252) ccw projected
  arc A442 (-21.6746, 32.1456) -> (-21.8276, 28.585) centre (-0.8708, 29.4676) ccw projected
  arc A443 (-20.5122, 32.4797) -> (-21.6746, 32.1456) centre (0.3933, -42.4252) ccw projected
  arc A444 (-18.4915, 29.5441) -> (-20.5122, 32.4797) centre (-36.7173, 19.162) ccw projected
  arc A445 (-17.37, 29.8291) -> (-18.4915, 29.5441) centre (0.3933, -42.4252) ccw projected
  arc A446 (-16.9958, 33.3733) -> (-17.37, 29.8291) centre (3.6012, 29.4072) ccw projected
  arc A447 (-15.8149, 33.6345) -> (-16.9958, 33.3733) centre (0.3933, -42.4252) ccw projected
  arc A448 (-13.9807, 30.579) -> (-15.8149, 33.6345) centre (-32.8166, 21.35) ccw projected
  arc A449 (-12.8436, 30.7937) -> (-13.9807, 30.579) centre (0.3933, -42.4252) ccw projected
  arc A450 (-12.2498, 34.3077) -> (-12.8436, 30.7937) centre (8.0608, 29.0688) ccw projected
  arc A451 (-11.055, 34.495) -> (-12.2498, 34.3077) centre (0.3933, -42.4252) ccw projected
  arc A452 (-9.4142, 31.3314) -> (-11.055, 34.495) centre (-28.7875, 23.2913) ccw projected
  arc A453 (-8.266, 31.475) -> (-9.4142, 31.3314) centre (0.3933, -42.4252) ccw projected
  arc A454 (-7.4549, 34.9453) -> (-8.266, 31.475) centre (12.4907, 28.4538) ccw projected
  arc A455 (-6.2507, 35.058) -> (-7.4549, 34.9453) centre (0.3933, -42.4252) ccw projected
  arc A456 (-4.8098, 31.7984) -> (-6.2507, 35.058) centre (-24.6455, 24.9783) ccw projected
  arc A457 (-3.6549, 31.8704) -> (-4.8098, 31.7984) centre (0.3933, -42.4252) ccw projected
  arc A458 (-2.6296, 35.2835) -> (-3.6549, 31.8704) centre (16.8738, 27.5646) ccw projected
  arc A459 (-1.4208, 35.3212) -> (-2.6296, 35.2835) centre (0.3933, -42.4252) ccw projected
  arc A460 (-0.1853, 31.9783) -> (-1.4208, 35.3212) centre (-20.4066, 26.4046) ccw projected
  arc A461 (0.9719, 31.9783) -> (-0.1853, 31.9783) centre (0.3933, -42.4252) ccw projected
  arc A462 (2.2073, 35.3212) -> (0.9719, 31.9783) centre (21.1932, 26.4046) ccw projected
  arc A463 (3.4162, 35.2835) -> (2.2073, 35.3212) centre (0.3933, -42.4252) ccw projected
  arc A464 (4.4415, 31.8704) -> (3.4162, 35.2835) centre (-16.0873, 27.5646) ccw projected
  arc A465 (5.5964, 31.7984) -> (4.4415, 31.8704) centre (0.3933, -42.4252) ccw projected
  arc A466 (7.0373, 35.058) -> (5.5964, 31.7984) centre (25.4321, 24.9783) ccw projected
  arc A467 (8.2415, 34.9453) -> (7.0373, 35.058) centre (0.3933, -42.4252) ccw projected
  arc A468 (9.0525, 31.475) -> (8.2415, 34.9453) centre (-11.7041, 28.4538) ccw projected
  arc A469 (10.2008, 31.3314) -> (9.0525, 31.475) centre (0.3933, -42.4252) ccw projected
  arc A470 (11.8415, 34.495) -> (10.2008, 31.3314) centre (29.5741, 23.2913) ccw projected
  arc A471 (13.0364, 34.3077) -> (11.8415, 34.495) centre (0.3933, -42.4252) ccw projected
  arc A472 (13.6301, 30.7937) -> (13.0364, 34.3077) centre (-7.2742, 29.0688) ccw projected
  arc A473 (14.7672, 30.579) -> (13.6301, 30.7937) centre (0.3933, -42.4252) ccw projected
  arc A474 (16.6015, 33.6345) -> (14.7672, 30.579) centre (33.6032, 21.35) ccw projected
  arc A475 (17.7824, 33.3733) -> (16.6015, 33.6345) centre (0.3933, -42.4252) ccw projected
  arc A476 (18.1565, 29.8291) -> (17.7824, 33.3733) centre (-2.8146, 29.4072) ccw projected
  arc A477 (19.2781, 29.5441) -> (18.1565, 29.8291) centre (0.3933, -42.4252) ccw projected
  arc A478 (21.2987, 32.4797) -> (19.2781, 29.5441) centre (37.5039, 19.162) ccw projected
  arc A479 (22.4611, 32.1456) -> (21.2987, 32.4797) centre (0.3933, -42.4252) ccw projected
  arc A480 (22.6142, 28.585) -> (22.4611, 32.1456) centre (1.6574, 29.4676) ccw projected
  arc A481 (23.7158, 28.2308) -> (22.6142, 28.585) centre (0.3933, -42.4252) ccw projected
  arc A482 (25.9151, 31.0352) -> (23.7158, 28.2308) centre (41.2609, 16.7357) ccw projected
  arc A483 (27.0545, 30.6294) -> (25.9151, 31.0352) centre (0.3933, -42.4252) ccw projected
  arc A484 (26.9859, 27.0662) -> (27.0545, 30.6294) centre (6.1245, 29.25) ccw projected
  arc A485 (28.0634, 26.6442) -> (26.9859, 27.0662) centre (0.3933, -42.4252) ccw projected
  arc A486 (30.4328, 29.3064) -> (28.0634, 26.6442) centre (44.8599, 14.0806) ccw projected
  arc A487 (31.5447, 28.8305) -> (30.4328, 29.3064) centre (0.3933, -42.4252) ccw projected
  arc A488 (31.2547, 25.2785) -> (31.5447, 28.8305) centre (10.5694, 28.755) ccw projected
  arc A489 (32.3039, 24.7904) -> (31.2547, 25.2785) centre (0.3933, -42.4252) ccw projected
  arc A490 (34.8342, 27.3001) -> (32.3039, 24.7904) centre (48.2868, 11.2068) ccw projected
  arc A491 (35.9144, 26.756) -> (34.8342, 27.3001) centre (0.3933, -42.4252) ccw projected
  arc A492 (35.4041, 23.2289) -> (35.9144, 26.756) centre (14.975, 27.9847) ccw projected
  arc A493 (36.4209, 22.6765) -> (35.4041, 23.2289) centre (0.3933, -42.4252) ccw projected
  arc A494 (39.1023, 25.024) -> (36.4209, 22.6765) centre (51.5284, 8.1255) ccw projected
  arc A495 (40.1466, 24.4139) -> (39.1023, 25.024) centre (0.3933, -42.4252) ccw projected
  arc A496 (39.4181, 20.9253) -> (40.1466, 24.4139) centre (19.3241, 26.942) ccw projected
  arc A497 (40.3986, 20.3107) -> (39.4181, 20.9253) centre (0.3933, -42.4252) ccw projected
  arc A498 (43.2208, 22.487) -> (40.3986, 20.3107) centre (54.5722, 4.8487) ccw projected
  arc A499 (44.2251, 21.8131) -> (43.2208, 22.487) centre (0.3933, -42.4252) ccw projected
  arc A500 (43.2811, 18.3766) -> (44.2251, 21.8131) centre (23.6, 25.6308) ccw projected
  arc A501 (44.2215, 17.7022) -> (43.2811, 18.3766) centre (0.3933, -42.4252) ccw projected
  arc A502 (47.1735, 19.6989) -> (44.2215, 17.7022) centre (57.4064, 1.3889) ccw projected
  arc A503 (48.134, 18.9638) -> (47.1735, 19.6989) centre (0.3933, -42.4252) ccw projected
  arc A504 (46.9781, 15.5926) -> (48.134, 18.9638) centre (27.7862, 24.0564) ccw projected
  arc A505 (47.8748, 14.8611) -> (46.9781, 15.5926) centre (0.3933, -42.4252) ccw projected
  arc A506 (50.9452, 16.6704) -> (47.8748, 14.8611) centre (60.0201, -2.2403) ccw projected
  arc A507 (51.8581, 15.8771) -> (50.9452, 16.6704) centre (0.3933, -42.4252) ccw projected
  arc A508 (50.495, 12.5842) -> (51.8581, 15.8771) centre (31.8663, 22.2248) ccw projected
  arc A509 (51.3444, 11.7984) -> (50.495, 12.5842) centre (0.3933, -42.4252) ccw projected
  arc A510 (54.5214, 13.4133) -> (51.3444, 11.7984) centre (62.403, -6.025) ccw projected
  arc A511 (55.3832, 12.5647) -> (54.5214, 13.4133) centre (0.3933, -42.4252) ccw projected
  arc A512 (53.818, 9.363) -> (55.3832, 12.5647) centre (35.8247, 20.1431) ccw projected
  arc A513 (54.6169, 8.5259) -> (53.818, 9.363) centre (0.3933, -42.4252) ccw projected
  arc A514 (57.8881, 9.9401) -> (54.6169, 8.5259) centre (64.546, -9.9505) ccw projected
  arc A515 (58.6956, 9.0397) -> (57.8881, 9.9401) centre (0.3933, -42.4252) ccw projected
  arc A516 (56.9343, 5.9415) -> (58.6956, 9.0397) centre (39.646, 17.8193) ccw projected
  arc A517 (57.6796, 5.0563) -> (56.9343, 5.9415) centre (0.3933, -42.4252) ccw projected
  arc A518 (61.0324, 6.2644) -> (57.6796, 5.0563) centre (66.4409, -14.0017) ccw projected
  arc A519 (61.7823, 5.3155) -> (61.0324, 6.2644) centre (0.3933, -42.4252) ccw projected
  arc A520 (59.8318, 2.3328) -> (61.7823, 5.3155) centre (43.3155, 15.2625) ccw projected
  arc A521 (60.5207, 1.403) -> (59.8318, 2.3328) centre (0.3933, -42.4252) ccw projected
  arc A522 (63.9422, 2.4003) -> (60.5207, 1.403) centre (68.0802, -18.1629) ccw projected
  arc A523 (64.6316, 1.4066) -> (63.9422, 2.4003) centre (0.3933, -42.4252) ccw projected
  arc A524 (62.4994, -1.4491) -> (64.6316, 1.4066) centre (46.8189, 12.4824) ccw projected
  arc A525 (63.1292, -2.4199) -> (62.4994, -1.4491) centre (0.3933, -42.4252) ccw projected
  arc A526 (66.606, -1.6372) -> (63.1292, -2.4199) centre (69.4576, -22.4179) ccw projected
  arc A527 (67.2323, -2.6719) -> (66.606, -1.6372) centre (0.3933, -42.4252) ccw projected
  arc A528 (64.9268, -5.3895) -> (67.2323, -2.6719) centre (50.1426, 9.4899) ccw projected
  arc A529 (65.4949, -6.3976) -> (64.9268, -5.3895) centre (0.3933, -42.4252) ccw projected
  arc A530 (69.0137, -5.8325) -> (65.4949, -6.3976) centre (70.5679, -26.7503) ccw projected
  arc A531 (69.5745, -6.9041) -> (69.0137, -5.8325) centre (0.3933, -42.4252) ccw projected
  arc A532 (67.1044, -9.4731) -> (69.5745, -6.9041) centre (53.2739, 6.2966) ccw projected
  arc A533 (67.6088, -10.5146) -> (67.1044, -9.4731) centre (0.3933, -42.4252) ccw projected
  arc A534 (71.1559, -10.1694) -> (67.6088, -10.5146) centre (71.4066, -31.1433) ccw projected
  arc A535 (71.649, -11.2738) -> (71.1559, -10.1694) centre (0.3933, -42.4252) ccw projected
  arc A536 (69.024, -13.6843) -> (71.649, -11.2738) centre (56.2007, 2.9148) ccw projected
  arc A537 (69.4627, -14.7551) -> (69.024, -13.6843) centre (0.3933, -42.4252) ccw projected
  arc A538 (73.0244, -14.6311) -> (69.4627, -14.7551) centre (71.9707, -35.58) ccw projected
  arc A539 (73.4478, -15.764) -> (73.0244, -14.6311) centre (0.3933, -42.4252) ccw projected
  arc A540 (70.6781, -18.0066) -> (73.4478, -15.764) centre (58.9115, -0.6424) ccw projected
  arc A541 (71.0493, -19.1026) -> (70.6781, -18.0066) centre (0.3933, -42.4252) ccw projected
  arc A542 (74.6118, -19.2003) -> (71.0493, -19.1026) centre (72.2578, -40.0432) ccw projected
  arc A543 (74.964, -20.3574) -> (74.6118, -19.2003) centre (0.3933, -42.4252) ccw projected
  arc A544 (72.0602, -22.4234) -> (74.964, -20.3574) centre (61.3959, -4.3613) ccw projected
  arc A545 (72.3626, -23.5404) -> (72.0602, -22.4234) centre (0.3933, -42.4252) ccw projected
  arc A546 (75.9121, -23.8594) -> (72.3626, -23.5404) centre (72.2668, -44.5156) ccw projected
  arc A547 (76.1917, -25.0361) -> (75.9121, -23.8594) centre (0.3933, -42.4252) ccw projected
  arc A548 (73.1651, -26.9176) -> (76.1917, -25.0361) centre (63.6443, -8.2275) ccw projected
  arc A549 (73.3974, -28.0512) -> (73.1651, -26.9176) centre (0.3933, -42.4252) ccw projected
  arc A550 (76.9203, -28.5903) -> (73.3974, -28.0512) centre (71.9978, -48.9799) ccw projected
  arc A551 (77.1262, -29.7821) -> (76.9203, -28.5903) centre (0.3933, -42.4252) ccw projected
  arc A552 (73.9884, -31.4718) -> (77.1262, -29.7821) centre (65.648, -12.2259) ccw projected
  arc A553 (74.1498, -32.6177) -> (73.9884, -31.4718) centre (0.3933, -42.4252) ccw projected
  arc A554 (77.6324, -33.3747) -> (74.1498, -32.6177) centre (71.4518, -53.4189) ccw projected
  arc A555 (77.7638, -34.577) -> (77.6324, -33.3747) centre (0.3933, -42.4252) ccw projected
  arc A556 (74.527, -36.0684) -> (77.7638, -34.577) centre (67.3993, -16.3412) ccw projected
  arc A557 (74.6169, -37.2221) -> (74.527, -36.0684) centre (0.3933, -42.4252) ccw projected
  arc A558 (78.0456, -38.1941) -> (74.6169, -37.2221) centre (70.6309, -57.8153) ccw projected
  arc A559 (78.102, -39.4023) -> (78.0456, -38.1941) centre (0.3933, -42.4252) ccw projected
  arc A560 (74.7788, -40.6896) -> (78.102, -39.4023) centre (68.8913, -20.5574) ccw projected
  arc A561 (74.7968, -41.8466) -> (74.7788, -40.6896) centre (0.3933, -42.4252) ccw projected
  arc A562 (78.1584, -43.0299) -> (74.7968, -41.8466) centre (69.5382, -62.1521) ccw projected
  arc A563 (78.1396, -44.2392) -> (78.1584, -43.0299) centre (0.3933, -42.4252) ccw projected
  arc A564 (74.7428, -45.3174) -> (78.1396, -44.2392) centre (70.1183, -24.8582) ccw projected
  arc A565 (74.6888, -46.4734) -> (74.7428, -45.3174) centre (0.3933, -42.4252) ccw projected
  arc A566 (77.9704, -47.8634) -> (74.6888, -46.4734) centre (68.1781, -66.4127) ccw projected
  arc A567 (77.8765, -49.0692) -> (77.9704, -47.8634) centre (0.3933, -42.4252) ccw projected
  arc A568 (74.4192, -49.9341) -> (77.8765, -49.0692) centre (71.0756, -29.2269) ccw projected
  arc A569 (74.2934, -51.0845) -> (74.4192, -49.9341) centre (0.3933, -42.4252) ccw projected
  arc A570 (77.4823, -52.6758) -> (74.2934, -51.0845) centre (66.5557, -70.5805) ccw projected
  arc A571 (77.3135, -53.8734) -> (77.4823, -52.6758) centre (0.3933, -42.4252) ccw projected
  arc A572 (73.8091, -54.5218) -> (77.3135, -53.8734) centre (71.7594, -33.6468) ccw projected
  arc A573 (73.6121, -55.6621) -> (73.8091, -54.5218) centre (0.3933, -42.4252) ccw projected
  arc A574 (76.6959, -57.4486) -> (73.6121, -55.6621) centre (64.6773, -74.6393) ccw projected
  arc A575 (76.453, -58.6334) -> (76.6959, -57.4486) centre (0.3933, -42.4252) ccw projected
  arc A576 (72.9151, -59.0626) -> (76.453, -58.6334) centre (72.1671, -38.1006) ccw projected
  arc A577 (72.6476, -60.1884) -> (72.9151, -59.0626) centre (0.3933, -42.4252) ccw projected
  arc A578 (75.6143, -62.1632) -> (72.6476, -60.1884) centre (62.5502, -78.5735) ccw projected
  arc A579 (75.2982, -63.3307) -> (75.6143, -62.1632) centre (0.3933, -42.4252) ccw projected
  arc A580 (71.7405, -63.5391) -> (75.2982, -63.3307) centre (72.2971, -42.5711) ccw projected
  arc A581 (71.4035, -64.6461) -> (71.7405, -63.5391) centre (0.3933, -42.4252) ccw projected
  arc A582 (74.2417, -66.8015) -> (71.4035, -64.6461) centre (60.1826, -82.3678) ccw projected
  arc A583 (73.8536, -67.947) -> (74.2417, -66.8015) centre (0.3933, -42.4252) ccw projected
  arc A584 (70.2898, -67.9339) -> (73.8536, -67.947) centre (72.1489, -47.041) ccw projected
  arc A585 (69.8846, -69.0178) -> (70.2898, -67.9339) centre (0.3933, -42.4252) ccw projected